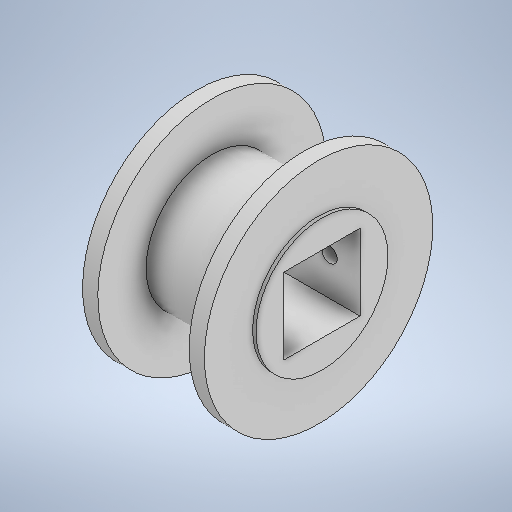
# Autodesk Inventor part: Pieza 8
Saved by Autodesk Inventor 2025.3 (Build 293356030, 356C)
## iProperties
Created: 2025-08-24
Part Number: Pieza 8
Material: Generic
Document SubType Name: Modeling
Designer: PC
Density: 1 g/cm^3
Appearance: Default
Author: PC
Autodesk Inventor part; units mm, degrees
ref_plane "YZ Plane" through (0, 0, 0) normal (1, 0, 0) x (0, 1, 0)
ref_plane "XZ Plane" through (0, 0, 0) normal (0, 1, 0) x (-1, 0, 0)
ref_plane "XY Plane" through (0, 0, 0) normal (0, 0, 1) x (1, 0, 0)
sketch "Sketch1" plane through (0, 0, 0) normal (0, 0, 1) x (1, 0, 0)
  line L0 (-9, 0) -> (-9, 7.2)
  line L1 (-9, 7.2) -> (-9.6665, 7.2)
  line L2 (-9.6665, 7.2) -> (-9.6665, 16.7)
  line L3 (-9.6665, 16.7) -> (-12.6665, 16.7)
  line L4 (-12.6665, 16.7) -> (-12.6665, 9.4)
  line L5 (-35, 0) -> (-35, 7.2)
  line L6 (-35, 7.2) -> (-33.6665, 7.2)
  line L7 (-33.6665, 7.2) -> (-33.6665, 16.7)
  line L8 (-33.6665, 16.7) -> (-30.6665, 16.7)
  line L9 (-30.6665, 16.7) -> (-30.6665, 7.2)
  line L10 (-41.0656, -5.8) -> (-47.8962, -5.8)
  line L11 (-12.6665, 9.4) -> (-12.6665, 7.2)
  line L12 (-30.6665, 7.2) -> (-12.6665, 7.2)
  line L13 (-35, 0) -> (-35, -5.8)
  line L14 (-9, 0) -> (-9, -5.8)
  line L15 (-9, -5.8) -> (-35, -5.8)
  circle A0 centre (-15, -5.8) radius 1.5
  point P0 (0, 0)
  point P1 (-16.5, -5.8)
  point P2 (-13.5, -5.8)
  dimension "d5" = 3
  dimension "d6" = 45
  dimension "d7" = 26
  dimension "d9" = 3
  dimension "d11" = 18
  dimension "d12" = 26
  constraints: 32 end point, 5 vertical, 3 horizontal, 2 perpendicular, 1 centre point, 1 point on line
  measures "d5" distance of L7.end L8.end
  measures "d6" diameter of L8 L10
  measures "d7" diameter of L6.end L10
  measures "d9" diameter of A0
  measures "d11" distance of L3.end L8.end
  measures "d12" distance of L13.end L14.end
revolve "Revolution1" add sketch "Sketch1" angle 360 about axis through (-41.0656, -5.8, 0) along (-1, 0, 0) contours L14 L15 A0 L13 L5 L6 L7 L8 L9 L12 L11 L4 L3 L2 L1 L0
sketch "Sketch2" plane through (-9, -5.8, 0) normal (1, 0, 0) x (0, 0, -1)
  line L0 (7.5, -7.5) -> (-7.5, -7.5)
  line L1 (-7.5, -7.5) -> (-7.5, 7.5)
  line L2 (-7.5, 7.5) -> (7.5, 7.5)
  line L3 (7.5, 7.5) -> (7.5, -7.5)
  line L4 (7.5, -7.5) -> (-7.5, 7.5) construction
  line L5 (-7.5, -7.5) -> (7.5, 7.5) construction
  point P0 (0, 5.8)
  point P1 (0, 0)
  dimension "d14" = 15
  dimension "d15" = 15
  constraints: 12 end point, 2 midpoint, 2 parallel, 1 horizontal, 1 perpendicular
  measures "d14" distance of L1.end L2.end
  measures "d15" distance of L0.end L1.end
extrude "Extrusion1" cut sketch "Sketch2" against normal blind 100
extrude "Extrusion2" cut sketch "Sketch1" along normal mid plane 100 contours A0 L15 | L15 A0
body "Solid1"
